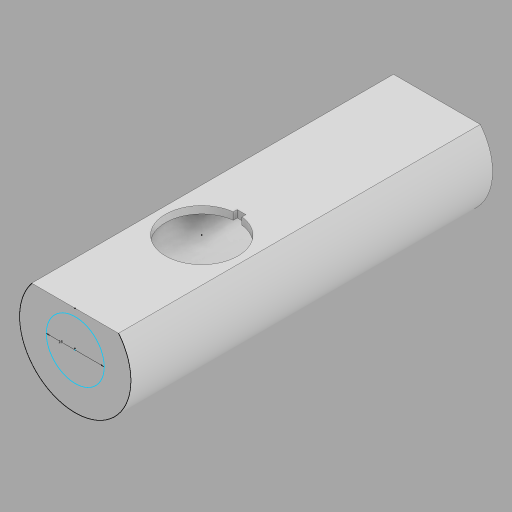
# Autodesk Inventor part: fleshlight
Saved by Autodesk Inventor 2024 (Build 280153000, 153)
## iProperties
Created: 2025-04-09
Part Number: fleshlight
Material: Generic
Document SubType Name: Modeling
Designer: lundm
Density: 1 g/cm^3
Appearance: Default
Author: lundm
Autodesk Inventor part; units mm, degrees
ref_plane "YZ Plane" through (0, 0, 0) normal (1, 0, 0) x (0, 1, 0)
ref_plane "XZ Plane" through (0, 0, 0) normal (0, 1, 0) x (-1, 0, 0)
ref_plane "XY Plane" through (0, 0, 0) normal (0, 0, 1) x (1, 0, 0)
sketch "Sketch1" plane through (0, 0, 0) normal (0, 1, 0) x (-1, 0, 0)
  arc A0 (1.2, -9.9277) -> (-1.2, -9.9277) centre (0, 0) ccw
  line L0 (0, 10) -> (21, 10) construction
  line L1 (0, -11) -> (-1.2, -11)
  line L2 (-1.2, -11) -> (-1.2, -9.9277)
  line L3 (0, -11) -> (1.2, -11)
  line L4 (0, -11) -> (1.2, -11) construction
  line L5 (1.2, -11) -> (1.2, -9.9277)
  dimension "d0" = 20
  dimension "d1" = 21
  dimension "d3" = 1.2
  dimension "d4" = 1.2
  dimension "d5" = 0
  constraints: 12 end point, 3 perpendicular, 3 point on circle, 2 horizontal, 1 centre point, 1 coincident, 1 collinear
  measures "d0" diameter of A0
  measures "d1" distance of L0.start L1.start
  measures "d3" distance of L1.start L1.end
  measures "d4" distance of L1.start L3.end
  measures "d5" distance between parallel lines of L3 L4
sketch "Sketch2" plane through (0, 0, 0) normal (1, 0, 0) x (0, 1, 0)
  point P0 (0, 0)
sketch "Sketch3" plane through (0, 0, 0) normal (0, 0, 1) x (1, 0, 0)
  line L0 (0, 0) -> (0, -22.8)
  line L1 (0, 0) -> (22.8, 0) construction
  line L2 (-10, 0) -> (-12, 0)
  line L3 (-10, 0) -> (-8, 0) construction
  line L4 (0, -22.8) -> (0, -25)
  line L5 (0, -22.8) -> (2.2, -22.8) construction
  arc A0 (-12, 0) -> (12, 0) centre (0, -9.62) ccw
  line L6 (12, 0) -> (10, 0)
  line L7 (12, 0) -> (14, 0) construction
  line L8 (-12, 0) -> (12, 0)
  dimension "d7" = 22.8
  dimension "d8" = 90
  dimension "d10" = 2
  dimension "d11" = 180
  dimension "d12" = 2.2
  dimension "d13" = 90
  dimension "d14" = 2
  dimension "d15" = 180
  constraints: 18 end point, 5 horizontal, 4 equal length, 3 point on circle, 2 collinear, 2 point on line, 2 vertical, 1 centre point
  measures "d7" distance of L0.start L0.end
  measures "d8" angle of L0 L1
  measures "d10" distance of L2.start L2.end
  measures "d11" angle of L2 L3
  measures "d12" distance of L0.end L4.end
  measures "d13" angle of L4 L5
  measures "d14" distance of L6.start L6.end
  measures "d15" angle of L6 L7
extrude "Extrusion1" add sketch "Sketch3" along normal blind 35 and the other way blind 65
shell "Shell1" thickness 2 removed faces 0
extrude "Extrusion2" cut sketch "Sketch1" against normal up to next
sketch "Sketch4" plane through (0, 0, 35) normal (0, 0, 1) x (1, 0, 0)
  arc A0 (-12, 0) -> (12, 0) centre (0, -9.62) ccw projected
  circle A1 centre (0, -10) radius 8
  point P0 (0, 0)
  dimension "d23" = 16
  constraints: 1 centre point
  measures "d23" diameter of A1
body "Solid1"
